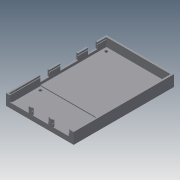
# Autodesk Inventor part: raspi_enclosure
Saved by Autodesk Inventor 2015 (Build 190159000, 159)
## iProperties
Created: 2018-01-14
Part Number: raspi_enclosure
Material: Generic
Document SubType Name: Modeling
Designer: rissa
Density: 1 g/cm^3
Appearance: Default
Author: rissa
Autodesk Inventor part; units mm, degrees
ref_plane "YZ Plane" through (0, 0, 0) normal (1, 0, 0) x (0, 1, 0)
ref_plane "XZ Plane" through (0, 0, 0) normal (0, 1, 0) x (-1, 0, 0)
ref_plane "XY Plane" through (0, 0, 0) normal (0, 0, 1) x (1, 0, 0)
sketch "Sketch1" plane through (0, 0, 0) normal (0, 1, 0) x (-1, 0, 0)
  line L0 (89.3441, 14.7035) -> (28.3441, 14.7035)
  line L1 (28.3441, 14.7035) -> (28.3441, -75.7965)
  line L2 (28.3441, -75.7965) -> (89.3441, -75.7965)
  line L3 (89.3441, -75.7965) -> (89.3441, 14.7035)
  point P0 (0, 0)
  dimension "d0" = 90.5
  dimension "d1" = 61
  constraints: 8 end point, 2 parallel, 1 horizontal, 1 perpendicular
  measures "d0" distance of L0.end L1.end
  measures "d1" distance of L1.end L2.end
extrude "Extrusion1" add sketch "Sketch1" along normal blind 1.5
sketch "Sketch2" plane through (0, 1.5, 0) normal (0, 1, 0) x (1, 0, 0)
  line L0 (-87.8441, -13.7035) -> (-29.8441, -13.7035)
  line L1 (-29.8441, -13.7035) -> (-29.8441, 74.2965)
  line L2 (-29.8441, 74.2965) -> (-87.8441, 74.2965)
  line L3 (-87.8441, 74.2965) -> (-87.8441, -13.7035)
  line L4 (-28.3441, 75.7965) -> (-89.3441, 75.7965) projected
  line L5 (-89.3441, -14.7035) -> (-28.3441, -14.7035) projected
  line L6 (-28.3441, -14.7035) -> (-28.3441, 75.7965) projected
  line L7 (-89.3441, 75.7965) -> (-89.3441, -14.7035) projected
  point P0 (0, 0)
  dimension "d4" = 1.5
  dimension "d5" = 1
  dimension "d6" = 1.5
  dimension "d7" = 1.5
  constraints: 8 end point, 2 parallel, 1 horizontal, 1 perpendicular
  measures "d4" distance between parallel lines of L4 L2
  measures "d5" distance between parallel lines of L5 L0
  measures "d6" distance between parallel lines of L1 L6
  measures "d7" distance between parallel lines of L7 L3
extrude "Extrusion2" add sketch "Sketch2" along normal blind 8.5
sketch "Sketch3" plane through (-89.3441, 0, 14.7035) normal (0, 0, 1) x (1, 0, 0)
  line L0 (61, 0) -> (61, 10) projected
  line L1 (0, 0) -> (0, 10) projected
  line L2 (59.5, 1.5) -> (59.5, 10) projected
  line L3 (1.5, 1.5) -> (1.5, 10) projected
  line L4 (0, 0) -> (61, 0) projected
  line L5 (1.5, 1.5) -> (59.5, 1.5) projected
  line L6 (0, 10) -> (61, 10) projected
  line L7 (42.5, 10) -> (56.5, 10)
  line L8 (56.5, 10) -> (56.5, 1.5)
  line L9 (56.5, 1.5) -> (42.5, 1.5)
  line L10 (42.5, 1.5) -> (42.5, 10)
  line L11 (24, 10) -> (38, 10)
  line L12 (38, 10) -> (38, 1.5)
  line L13 (38, 1.5) -> (24, 1.5)
  line L14 (24, 1.5) -> (24, 10)
  line L15 (3.5, 10) -> (20.5, 10)
  line L16 (20.5, 10) -> (20.5, 1.5)
  line L17 (20.5, 1.5) -> (3.5, 1.5)
  line L18 (3.5, 1.5) -> (3.5, 10)
  point P0 (89.3441, 0)
  dimension "d10" = 61
  dimension "d11" = 58
  dimension "d12" = 1.5
  dimension "d13" = 10
  dimension "d14" = 3
  dimension "d15" = 14
  dimension "d16" = 14
  dimension "d17" = 4.5
  dimension "d18" = 3.5
  dimension "d19" = 17
  dimension "d20" = 2
  constraints: 24 end point, 6 parallel, 6 point on line, 3 horizontal, 3 perpendicular
  measures "d10" distance between parallel lines of L0 L1
  measures "d11" distance between parallel lines of L2 L3
  measures "d12" distance between parallel lines of L4 L5
  measures "d13" distance between parallel lines of L4 L6
  measures "d14" distance between parallel lines of L2 L8
  measures "d15" distance between parallel lines of L8 L10
  measures "d16" distance between parallel lines of L12 L14
  measures "d17" distance between parallel lines of L10 L12
  measures "d18" distance between parallel lines of L14 L16
  measures "d19" distance between parallel lines of L16 L18
  measures "d20" distance between parallel lines of L18 L3
extrude "Extrusion3" cut sketch "Sketch3" against normal blind 2 contours L8 L5 L10 L6 | L6 L16 L5 L18 | L12 L5 L14 L6
sketch "Sketch4" plane through (-89.3441, 0, -75.7965) normal (-1, 0, 0) x (0, 0, 1)
  line L0 (90.5, 0) -> (90.5, 10) projected
  line L1 (0, 0) -> (0, 10) projected
  line L2 (89.5, 1.5) -> (89.5, 10) projected
  line L3 (1.5, 1.5) -> (1.5, 10) projected
  line L4 (0, 0) -> (90.5, 0) projected
  line L5 (1.5, 1.5) -> (89.5, 1.5) projected
  line L6 (0, 10) -> (90.5, 10) projected
  line L7 (61, 10) -> (53, 10)
  line L8 (53, 10) -> (53, 1.5)
  line L9 (53, 1.5) -> (61, 1.5)
  line L10 (61, 1.5) -> (61, 10)
  line L11 (89.5, 10) -> (1.5, 10) projected
  line L12 (89.5, 1.5) -> (1.5, 1.5) projected
  line L13 (27, 10) -> (43, 10)
  line L14 (43, 10) -> (43, 1.5)
  line L15 (43, 1.5) -> (27, 1.5)
  line L16 (27, 1.5) -> (27, 10)
  line L17 (9.5, 10) -> (18, 10)
  line L18 (18, 10) -> (18, 1.5)
  line L19 (18, 1.5) -> (9.5, 1.5)
  line L20 (9.5, 1.5) -> (9.5, 10)
  point P0 (75.7965, 0)
  dimension "d23" = 90.5
  dimension "d24" = 88
  dimension "d25" = 1.5
  dimension "d26" = 10
  dimension "d27" = 28.5
  dimension "d28" = 8
  dimension "d29" = 10
  dimension "d30" = 16
  dimension "d31" = 9
  dimension "d32" = 8.5
  dimension "d33" = 8
  constraints: 24 end point, 6 parallel, 6 point on line, 3 horizontal, 3 perpendicular
  measures "d23" distance between parallel lines of L0 L1
  measures "d24" distance between parallel lines of L2 L3
  measures "d25" distance between parallel lines of L4 L5
  measures "d26" distance between parallel lines of L4 L6
  measures "d27" distance between parallel lines of L2 L10
  measures "d28" distance between parallel lines of L10 L8
  measures "d29" distance between parallel lines of L8 L14
  measures "d30" distance between parallel lines of L14 L16
  measures "d31" distance between parallel lines of L16 L18
  measures "d32" distance between parallel lines of L18 L20
  measures "d33" distance between parallel lines of L3 L20
extrude "Extrusion4" cut sketch "Sketch4" against normal blind 2 contours L10 L5 L8 L6 | L6 L18 L5 L20 | L14 L5 L16 L6
sketch "Sketch5" plane through (0, 10, 0) normal (0, 1, 0) x (1, 0, 0)
  line L0 (-29.8441, -13.7035) -> (-32.8441, -13.7035) projected
  line L1 (-32.8441, -14.7035) -> (-28.3441, -14.7035) projected
  line L2 (-28.3441, -14.7035) -> (-28.3441, 75.7965) projected
  line L3 (-32.8441, -13.7035) -> (-32.8441, -14.7035) projected
  line L4 (-32.8441, -14.7035) -> (-32.8441, -13.7035) projected
  line L5 (-89.3441, -14.7035) -> (-28.3441, -14.7035) projected
  line L6 (-32.8441, -14.2035) -> (-31.8441, -14.2035)
  line L7 (-31.8441, -14.2035) -> (-31.8441, -14.7035)
  line L8 (-31.8441, -14.7035) -> (-32.8441, -14.7035)
  line L9 (-32.8441, -14.7035) -> (-32.8441, -14.2035)
  point P0 (0, 0)
  dimension "d36" = 1
  dimension "d37" = 4.5
  dimension "d38" = 0.5
  dimension "d39" = 1
  constraints: 8 end point, 2 parallel, 1 horizontal, 1 midpoint, 1 perpendicular, 1 point on line
  measures "d36" distance between parallel lines of L0 L1
  measures "d37" distance between parallel lines of L2 L3
  measures "d38" distance between parallel lines of L1 L6
  measures "d39" distance of L6.end L6.start
extrude "Extrusion5" cut sketch "Sketch5" against normal blind 3
sketch "Sketch6" plane through (0, 10, 0) normal (0, 1, 0) x (1, 0, 0)
  line L0 (-51.3441, -14.7035) -> (-46.8441, -14.7035) projected
  line L1 (-46.8441, -13.7035) -> (-51.3441, -13.7035) projected
  line L2 (-46.8441, -14.7035) -> (-46.8441, -13.7035) projected
  line L3 (-51.3441, -14.7035) -> (-51.3441, -13.7035) projected
  line L4 (-46.8441, -14.2035) -> (-47.8441, -14.2035)
  line L5 (-47.8441, -14.2035) -> (-47.8441, -14.7035)
  line L6 (-47.8441, -14.7035) -> (-46.8441, -14.7035)
  line L7 (-46.8441, -14.7035) -> (-46.8441, -14.2035)
  point P0 (0, 0)
  dimension "d42" = 1
  dimension "d43" = 4.5
  dimension "d44" = 0.5
  dimension "d45" = 1
  constraints: 8 end point, 2 parallel, 1 horizontal, 1 midpoint, 1 perpendicular, 1 point on line
  measures "d42" distance between parallel lines of L0 L1
  measures "d43" distance between parallel lines of L2 L3
  measures "d44" distance between parallel lines of L0 L4
  measures "d45" distance between parallel lines of L5 L2
extrude "Extrusion6" cut sketch "Sketch6" against normal blind 3 contours L5 L4 L2 L0
sketch "Sketch7" plane through (0, 10, 0) normal (0, 1, 0) x (1, 0, 0)
  line L0 (-46.8441, -13.7035) -> (-51.3441, -13.7035) projected
  line L1 (-51.3441, -14.7035) -> (-47.8441, -14.7035) projected
  line L2 (-46.8441, -14.2035) -> (-46.8441, -13.7035) projected
  line L3 (-51.3441, -13.7035) -> (-51.3441, -14.7035) projected
  line L4 (-46.8441, -14.7035) -> (-47.8441, -14.7035) projected
  line L5 (-47.8441, -14.2035) -> (-46.8441, -14.2035) projected
  line L6 (-51.3441, -14.2035) -> (-50.3441, -14.2035)
  line L7 (-50.3441, -14.2035) -> (-50.3441, -14.7035)
  line L8 (-50.3441, -14.7035) -> (-51.3441, -14.7035)
  line L9 (-51.3441, -14.7035) -> (-51.3441, -14.2035)
  point P0 (0, 0)
  dimension "d48" = 1
  dimension "d49" = 4.5
  dimension "d50" = 0.5
  dimension "d51" = 0.5
  dimension "d52" = 1
  constraints: 8 end point, 2 parallel, 1 horizontal, 1 midpoint, 1 perpendicular, 1 point on line
  measures "d48" distance between parallel lines of L0 L1
  measures "d49" distance between parallel lines of L2 L3
  measures "d50" distance between parallel lines of L4 L5
  measures "d51" distance between parallel lines of L1 L6
  measures "d52" distance between parallel lines of L7 L3
extrude "Extrusion7" cut sketch "Sketch7" against normal blind 3
sketch "Sketch8" plane through (0, 10, 0) normal (0, 1, 0) x (1, 0, 0)
  line L0 (-65.3441, -13.7035) -> (-68.8441, -13.7035) projected
  line L1 (-68.8441, -14.7035) -> (-65.3441, -14.7035) projected
  line L2 (-68.8441, -13.7035) -> (-68.8441, -14.7035) projected
  line L3 (-65.3441, -14.7035) -> (-65.3441, -13.7035) projected
  line L4 (-65.3441, -14.7035) -> (-65.3441, -13.7035) projected
  line L5 (-65.3441, -14.2035) -> (-66.3441, -14.2035)
  line L6 (-66.3441, -14.2035) -> (-66.3441, -14.7035)
  line L7 (-66.3441, -14.7035) -> (-65.3441, -14.7035)
  line L8 (-65.3441, -14.7035) -> (-65.3441, -14.2035)
  point P0 (0, 0)
  dimension "d55" = 1
  dimension "d56" = 3.5
  dimension "d57" = 1
  dimension "d58" = 0.5
  constraints: 8 end point, 2 parallel, 1 horizontal, 1 midpoint, 1 perpendicular, 1 point on line
  measures "d55" distance between parallel lines of L0 L1
  measures "d56" distance between parallel lines of L2 L3
  measures "d57" distance between parallel lines of L6 L3
  measures "d58" distance between parallel lines of L1 L5
extrude "Extrusion8" cut sketch "Sketch8" against normal blind 3 contours L3 L1 L6 L5
sketch "Sketch9" plane through (-29.8441, 1.5, -74.2965) normal (-1, 0, 0) x (0, 0, 1)
  line L0 (0, 0) -> (0, 8.5) projected
  line L1 (0, 7.5) -> (88.9462, 7.5)
  line L2 (88.9462, 7.5) -> (88.9462, 6.5)
  line L3 (88.9462, 6.5) -> (0, 6.5)
  line L4 (0, 6.5) -> (0, 7.5)
  line L5 (0, 8.5) -> (88, 8.5) projected
  point P0 (74.2965, -1.5)
  dimension "d61" = 1
  dimension "d62" = 88.9462
  dimension "d63" = 1
  constraints: 8 end point, 2 parallel, 1 horizontal, 1 perpendicular, 1 point on line
  measures "d61" distance between parallel lines of L1 L3
  measures "d62" distance between parallel lines of L4 L2
  measures "d63" distance between parallel lines of L1 L5
extrude "Extrusion9" cut sketch "Sketch9" against normal blind 0.5
sketch "Sketch10" plane through (-87.8441, 1.5, 13.7035) normal (1, 0, 0) x (0, 0, -1)
  line L0 (28.5, 0) -> (28.5, 8.5) projected
  line L1 (0, 7.5) -> (28.5, 7.5)
  line L2 (28.5, 7.5) -> (28.5, 6.5)
  line L3 (28.5, 6.5) -> (0, 6.5)
  line L4 (0, 6.5) -> (0, 7.5)
  line L5 (0, 8.5) -> (28.5, 8.5) projected
  point P0 (13.7035, -1.5)
  dimension "d66" = 28.5
  dimension "d67" = 1
  dimension "d68" = 1
  constraints: 8 end point, 2 parallel, 1 horizontal, 1 perpendicular, 1 point on line
  measures "d66" distance of L1.start L1.end
  measures "d67" distance between parallel lines of L1 L3
  measures "d68" distance between parallel lines of L1 L5
extrude "Extrusion10" cut sketch "Sketch10" against normal blind 0.5
sketch "Sketch11" plane through (-87.8441, 1.5, -22.7965) normal (1, 0, 0) x (0, 0, -1)
  line L0 (0, 8.5) -> (0, 0) projected
  line L1 (10, 0) -> (10, 8.5) projected
  line L2 (0, 7.5) -> (10, 7.5)
  line L3 (10, 7.5) -> (10, 6.5)
  line L4 (10, 6.5) -> (0, 6.5)
  line L5 (0, 6.5) -> (0, 7.5)
  line L6 (0, 8.5) -> (10, 8.5) projected
  point P0 (-22.7965, -1.5)
  dimension "d71" = 10
  dimension "d72" = 1
  dimension "d73" = 1
  constraints: 8 end point, 2 parallel, 2 point on line, 1 horizontal, 1 perpendicular
  measures "d71" distance of L2.start L2.end
  measures "d72" distance between parallel lines of L4 L2
  measures "d73" distance between parallel lines of L2 L6
extrude "Extrusion11" cut sketch "Sketch11" against normal blind 0.5 contours L2 L1 L4 L0
sketch "Sketch12" plane through (-87.8441, 1.5, -48.7965) normal (1, 0, 0) x (0, 0, -1)
  line L0 (0, 8.5) -> (0, 0) projected
  line L1 (9, 0) -> (9, 8.5) projected
  line L2 (0, 7.5) -> (9, 7.5)
  line L3 (9, 7.5) -> (9, 6.5)
  line L4 (9, 6.5) -> (0, 6.5)
  line L5 (0, 6.5) -> (0, 7.5)
  line L6 (0, 8.5) -> (9, 8.5) projected
  point P0 (-48.7965, -1.5)
  dimension "d76" = 1
  dimension "d77" = 1
  constraints: 8 end point, 2 parallel, 2 point on line, 1 horizontal, 1 perpendicular
  measures "d76" distance between parallel lines of L6 L2
  measures "d77" distance between parallel lines of L4 L2
extrude "Extrusion12" cut sketch "Sketch12" against normal blind 0.5 contours L2 L1 L4 L0
sketch "Sketch13" plane through (-87.8441, 1.5, -74.2965) normal (1, 0, 0) x (0, 0, -1)
  line L0 (0, 0) -> (0, 8.5) projected
  line L1 (-8, 8.5) -> (-8, 0) projected
  line L2 (0, 7.5) -> (-8, 7.5)
  line L3 (-8, 7.5) -> (-8, 6.5)
  line L4 (-8, 6.5) -> (0, 6.5)
  line L5 (0, 6.5) -> (0, 7.5)
  line L6 (-8, 8.5) -> (0, 8.5) projected
  point P0 (-74.2965, -1.5)
  dimension "d80" = 1
  dimension "d81" = 1
  constraints: 8 end point, 2 parallel, 2 point on line, 1 horizontal, 1 perpendicular
  measures "d80" distance between parallel lines of L2 L4
  measures "d81" distance between parallel lines of L6 L2
extrude "Extrusion13" cut sketch "Sketch13" against normal blind 0.5 contours L4 L1 L2 L0
sketch "Sketch16" plane through (0, 1.5, 0) normal (0, 1, 0) x (1, 0, 0)
  line L0 (-87.8539, 14.7789) -> (-29.8441, 14.7789)
  line L1 (-29.8441, 14.7789) -> (-29.8441, 74.2965)
  line L2 (-29.8441, 74.2965) -> (-87.8539, 74.2965)
  line L3 (-87.8539, 74.2965) -> (-87.8539, 14.7789)
  line L4 (-89.3441, 22.7965) -> (-87.8539, 22.7965)
  line L5 (-87.8539, 22.7965) -> (-87.8539, 14.7789)
  line L6 (-87.8539, 14.7789) -> (-89.3441, 14.7789)
  line L7 (-89.3441, 14.7789) -> (-89.3441, 22.7965)
  line L8 (-89.3441, 48.7965) -> (-87.8441, 48.7965)
  line L9 (-87.8441, 48.7965) -> (-87.8441, 32.7965)
  line L10 (-87.8441, 32.7965) -> (-89.3441, 32.7965)
  line L11 (-89.3441, 32.7965) -> (-89.3441, 48.7965)
  line L12 (-89.3441, 66.2965) -> (-87.8539, 66.2965)
  line L13 (-87.8539, 66.2965) -> (-87.8539, 57.7072)
  line L14 (-87.8539, 57.7072) -> (-89.3441, 57.7072)
  line L15 (-89.3441, 57.7072) -> (-89.3441, 66.2965)
  line L16 (-89.3441, 66.2965) -> (-87.8539, 66.2965)
  line L17 (-87.8539, 66.2965) -> (-87.8539, 57.7072)
  line L18 (-87.8539, 57.7072) -> (-89.3441, 57.7072)
  line L19 (-89.3441, 57.7072) -> (-89.3441, 66.2965)
  line L20 (-85.8441, -13.7035) -> (-68.8441, -13.7035)
  line L21 (-68.8441, -13.7035) -> (-68.8441, -14.7035)
  line L22 (-68.8441, -14.7035) -> (-85.8441, -14.7035)
  line L23 (-85.8441, -14.7035) -> (-85.8441, -13.7035)
  line L24 (-65.3441, -13.7035) -> (-51.3441, -13.7035)
  line L25 (-51.3441, -13.7035) -> (-51.3441, -14.7035)
  line L26 (-51.3441, -14.7035) -> (-65.3441, -14.7035)
  line L27 (-65.3441, -14.7035) -> (-65.3441, -13.7035)
  line L28 (-46.8441, -13.7035) -> (-32.8441, -13.7035)
  line L29 (-32.8441, -13.7035) -> (-32.8441, -14.7035)
  line L30 (-32.8441, -14.7035) -> (-46.8441, -14.7035)
  line L31 (-46.8441, -14.7035) -> (-46.8441, -13.7035)
  point P0 (0, 0)
  constraints: 64 end point, 16 parallel, 8 horizontal, 8 perpendicular, 1 point on line
extrude "Extrusion16" add sketch "Sketch16" along normal blind 3 contours L6 L7 L4 L3 | L10 L11 L8 L3 | L3 L8 L9 L10 | L3 L14 L15 L12 | L20 L21 L22 L23 | L24 L25 L26 L27 | L28 L29 L30 L31
sketch "Sketch17" plane through (0, 1.5, 0) normal (0, 1, 0) x (1, 0, 0)
  line L0 (-87.8539, 14.7965) -> (-29.8441, 14.7965)
  line L1 (-29.8441, 14.7965) -> (-29.8441, 74.2965)
  line L2 (-29.8441, 74.2965) -> (-87.8539, 74.2965)
  line L3 (-87.8539, 74.2965) -> (-87.8539, 14.7965)
  point P0 (0, 0)
  constraints: 8 end point, 2 parallel, 1 horizontal, 1 perpendicular
extrude "Extrusion17" add sketch "Sketch17" along normal blind 0.75
hole "Hole1" at (-84.3441, 1.5, -11.2965) direction (0, -1, 0) diameter 2.5 end through all
hole "Hole2" at (-33.3441, 1.5, -11.1445) direction (0, -1, 0) diameter 2.5 end through all
hole "Hole3" at (-84.3441, 2.25, -70.7965) direction (0, -1, 0) diameter 2.5 end through all
hole "Hole4" at (-33.3441, 2.25, -70.7965) direction (0, -1, 0) diameter 2.5 end through all
body "Solid1"
